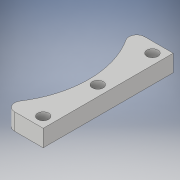
# Autodesk Inventor part: feeder_stack
Saved by Autodesk Inventor 2019 (Build 230136000, 136)
## iProperties
Created: 2018-11-15
Part Number: feeder_stack
Material: Generic
Document SubType Name: Modeling
Designer: chill
Density: 1 g/cm^3
Appearance: Default
Author: chill
Autodesk Inventor part; units mm, degrees
ref_plane "YZ Plane" through (0, 0, 0) normal (1, 0, 0) x (0, 1, 0)
ref_plane "XZ Plane" through (0, 0, 0) normal (0, 1, 0) x (-1, 0, 0)
ref_plane "XY Plane" through (0, 0, 0) normal (0, 0, 1) x (1, 0, 0)
sketch "Sketch1" plane through (0, 0, 0) normal (0, 1, 0) x (-1, 0, 0)
  arc A0 (-27.9508, 25) -> (-27.9508, -25) centre (0, 0) ccw
  line L0 (-27.9508, 25) -> (-45, 25)
  line L1 (-27.9508, -25) -> (-45, -25)
  line L2 (-45, 25) -> (-45, -25)
  circle A1 centre (-41, 21) radius 2.125
  circle A2 centre (-41, 0) radius 2.125
  circle A3 centre (-41, -21) radius 2.125
  dimension "d0" = 75
  dimension "d3" = 25
  dimension "d4" = 25
  dimension "d5" = 45
  dimension "d6" = 4.25
  dimension "d7" = 4.25
  dimension "d8" = 4.25
  dimension "d9" = 4
  dimension "d10" = 4
  dimension "d11" = 4
  dimension "d12" = 25
  dimension "d13" = 4
  dimension "d14" = 4
  constraints: 6 end point, 4 centre point, 2 horizontal, 2 point on circle, 1 coincident, 1 vertical
  measures "d0" diameter of A0
  measures "d3" distance from line of L0 point (0, 0)
  measures "d4" distance from line of L1 point (0, 0)
  measures "d5" distance from line of L2 point (0, 0)
  measures "d6" diameter of A1
  measures "d7" diameter of A2
  measures "d8" diameter of A3
  measures "d9" distance from line of L1 A3.centre
  measures "d10" distance from line of L2 A3.centre
  measures "d11" distance from line of L2 A2.centre
  measures "d12" distance from line of A2.centre L1
  measures "d13" distance from line of A1.centre L0
  measures "d14" distance from line of L2 A1.centre
extrude "Extrusion1" add sketch "Sketch1" along normal blind 6.5
fillet "Fillet1" radius 3 2 edges at (27.9508, 3.25, 25) (27.9508, 3.25, -25)
body "Solid1"
